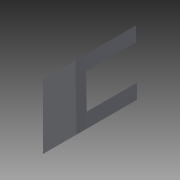
# Autodesk Inventor part: gimbal_stick_fixation
Saved by Autodesk Inventor 2015 SP1 (Build 190203100, 203)
## iProperties
Created: 2015-07-15
Part Number: gimbal_stick_fixation
Material: Generic
Document SubType Name: Modeling
Designer: Alexandre Cherpillod
Density: 1 g/cm^3
Appearance: Default
Author: Alexandre Cherpillod
Autodesk Inventor part; units mm, degrees
ref_plane "YZ Plane" through (0, 0, 0) normal (1, 0, 0) x (0, 1, 0)
ref_plane "XZ Plane" through (0, 0, 0) normal (0, 1, 0) x (-1, 0, 0)
ref_plane "XY Plane" through (0, 0, 0) normal (0, 0, 1) x (1, 0, 0)
sketch "Sketch2" plane through (0, 0, 0) normal (0, 1, 0) x (-1, 0, 0)
  line L0 (0, 0) -> (7.7547, -7.7547) construction
  line L1 (0, 0) -> (0, -11.6637) construction
  line L2 (-25.4458, 33.931) -> (0, 8.4853) construction
  line L3 (0, 0) -> (8, -8)
  line L4 (8, -11.5355) -> (8, -11.5355)
  line L5 (8, -8) -> (8, -11.5355)
  line L6 (0, 0) -> (0, -3.5355)
  line L7 (0, 8.4853) -> (0.2453, 8.24)
  line L8 (0.2453, 11.7755) -> (8, 4.0208)
  line L9 (8, 4.0208) -> (8, 0.4853)
  line L10 (0.2453, 8.24) -> (8, 0.4853)
  line L11 (8, -11.5355) -> (0, -3.5355)
  line L12 (0, 8.4853) -> (8, 0.4853) construction
  line L13 (0.2453, 8.24) -> (0.2453, 11.7755)
  dimension "d0" = 45
  dimension "d1" = 6
  dimension "d2" = 2.5
  dimension "d4" = 8
  constraints: 29 end point, 6 point on line, 4 parallel, 3 collinear, 3 vertical, 2 equal length
  measures "d0" angle of L0 L1
  measures "d1" distance between parallel lines of L0 L2
  measures "d2" distance between parallel lines of L0 L4
  measures "d4" horizontal distance of L4.end L6.end
extrude "Extrusion1" add sketch "Sketch2" along normal blind 12
sketch "Sketch3" plane through (0, 0, 0) normal (0, -1, 0) x (1, 0, 0)
  line L0 (-8, 4.0208) -> (-0.2453, 11.7755) projected
  line L1 (-8, -11.5355) -> (0, -3.5355) projected
  line L2 (-8, -8) -> (-8, -11.5355) projected
  line L3 (0, 26.3321) -> (0, -17.8468) projected
  line L4 (-8, 0.4853) -> (-8, 4.0208) projected
  line L5 (-0.2453, 11.7755) -> (0, -3.5355)
  line L6 (-8, -11.5355) -> (-8, 4.0208)
  line L7 (-8, 4.0208) -> (-0.2453, 11.7755)
  line L8 (0, -3.5355) -> (-8, -11.5355)
  point P0 (0, 0)
  point P1 (-15, -6.5147)
  constraints: 8 end point, 2 collinear, 1 vertical, 2 other
extrude "Extrusion2" add sketch "Sketch3" along normal blind 2.5
sketch "Sketch4" plane through (0, 0, 0) normal (0, 0, 1) x (1, 0, 0)
  line L0 (-8, 12) -> (-0.2453, 12) projected
  line L1 (-2.1227, 10) -> (-6.1227, 10)
  line L2 (-6.1227, 10) -> (-6.1227, 6)
  line L3 (-6.1227, 6) -> (-2.1227, 6)
  line L4 (-2.1227, 6) -> (-2.1227, 10)
  line L5 (-4.1227, 12) -> (-4.1227, 0)
  line L6 (0, 0) -> (-8, 0) projected
  point P0 (-4.1227, 10)
  dimension "d9" = 4
  dimension "d10" = 4
  dimension "d13" = 6
  constraints: 10 end point, 2 midpoint, 2 parallel, 1 horizontal, 1 perpendicular, 1 point on line, 1 vertical
  measures "d9" distance of L1.start L1.end
  measures "d10" distance of L1.end L2.end
  measures "d13" distance between parallel lines of L6 L3
extrude "Extrusion3" cut sketch "Sketch4" along normal through all both and the other way through all
body "Solid1"
